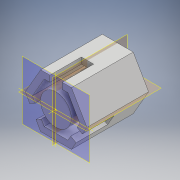
# Autodesk Inventor part: center
Saved by Autodesk Inventor 2017 (Build 210142000, 142)
## iProperties
Created: 2020-06-17
Part Number: center
Material: Generic
Document SubType Name: Modeling
Designer: HAYNIE R&D
Density: 1 g/cm^3
Appearance: Default
Author: HAYNIE R&D
Autodesk Inventor part; units mm, degrees
sketch "Sketch2" plane through (0, 0, 0) normal (0, 1, 0) x (-1, 0, 0)
  line L0 (-0.1126, -21.6377) -> (12.3874, -21.6377)
  line L1 (-0.1126, -21.6377) -> (-12.6126, -21.6377)
  line L2 (12.3874, -21.6377) -> (24.8874, 0.0129)
  line L3 (24.8874, 0.0129) -> (12.3874, 21.6635)
  line L4 (12.3874, 21.6635) -> (-12.6126, 21.6635)
  line L5 (-12.6126, 21.6635) -> (-25.1126, 0.0129)
  line L6 (-25.1126, 0.0129) -> (-12.6126, -21.6377)
  point P0 (0, 0)
  dimension "d12" = 12.5
  dimension "d13" = 12.5
  dimension "d14" = 25
  dimension "d15" = 25
  dimension "d16" = 120
  dimension "d17" = 25
  dimension "d18" = 25
  dimension "d19" = 120
  constraints: 14 end point, 3 horizontal, 1 parallel
  measures "d12" distance of L0.start L0.end
  measures "d13" distance of L0.start L1.end
  measures "d14" distance of L0.end L2.end
  measures "d15" distance of L2.end L3.end
  measures "d16" angle of L3 L2
  measures "d17" distance of L3.end L4.end
  measures "d18" distance of L4.end L5.end
  measures "d19" angle of L5 L4
extrude "Extrusion2" add sketch "Sketch2" along normal blind 50
shell "Shell1" thickness 5 removed faces 1 at (0.1126, 0, 7.2298)
sketch "Sketch3" plane through (-12.3874, 0, 21.6635) normal (0, 0, 1) x (1, 0, 0)
  line L0 (7.5, 25.4958) -> (17.5, 25.4958)
  line L1 (17.5, 25.4958) -> (17.5, -0.0042)
  line L2 (17.5, -0.0042) -> (7.5, -0.0042)
  line L3 (7.5, -0.0042) -> (7.5, 25.4958)
  line L4 (0, 0) -> (0, 50) projected
  point P0 (12.3874, 0)
  dimension "d23" = 25.5
  dimension "d24" = 10
  dimension "d25" = 7.5
  constraints: 8 end point, 2 parallel, 1 horizontal, 1 perpendicular
  measures "d23" distance of L0.end L1.end
  measures "d24" distance between parallel lines of L1 L3
  measures "d25" distance between parallel lines of L4 L3
extrude "Extrusion3" cut sketch "Sketch3" against normal blind 5
sketch "Sketch4" plane through (12.6126, 0, -21.6377) normal (0.8660254, 0, -0.5) x (-0.5, 0, -0.8660254)
  line L0 (-17.5, 25.4905) -> (-7.5, 25.4905)
  line L1 (-7.5, 25.4905) -> (-7.5, -0.0095)
  line L2 (-7.5, -0.0095) -> (-17.5, -0.0095)
  line L3 (-17.5, -0.0095) -> (-17.5, 25.4905)
  line L4 (-25, 0) -> (-25, 50) projected
  point P0 (-12.4325, 0)
  point P1 (12.3874, 0)
  dimension "d28" = 25.5
  dimension "d29" = 10
  dimension "d30" = 7.5
  constraints: 8 end point, 2 parallel, 1 horizontal, 1 perpendicular
  measures "d28" distance of L0.end L1.end
  measures "d29" distance between parallel lines of L1 L3
  measures "d30" distance between parallel lines of L3 L4
extrude "Extrusion4" cut sketch "Sketch4" against normal blind 5
sketch "Sketch5" plane through (-24.8874, 0, 0.0129) normal (-0.8660254, 0, -0.5) x (-0.5, 0, 0.8660254)
  line L0 (-17.5, 25.4996) -> (-7.5, 25.4996)
  line L1 (-7.5, 25.4996) -> (-7.5, -0.0004)
  line L2 (-7.5, -0.0004) -> (-17.5, -0.0004)
  line L3 (-17.5, -0.0004) -> (-17.5, 25.4996)
  line L4 (-25, 0) -> (-25, 50) projected
  point P0 (-12.4549, 0)
  point P1 (12.3874, 0)
  dimension "d33" = 25.5
  dimension "d34" = 10
  dimension "d35" = 7.5
  constraints: 8 end point, 2 parallel, 1 horizontal, 1 perpendicular
  measures "d33" distance of L0.end L1.end
  measures "d34" distance between parallel lines of L1 L3
  measures "d35" distance between parallel lines of L3 L4
extrude "Extrusion5" cut sketch "Sketch5" against normal blind 5
sketch "Sketch7" plane through (0, 50, 0) normal (0, 1, 0) x (1, 0, 0)
  circle A0 centre (0, 0) radius 12.5
  dimension "d39" = 25
  constraints: 1 centre point, 1 coincident
  measures "d39" diameter of A0
extrude "Extrusion6" add sketch "Sketch7" along normal blind 5 and the other way blind 50
hole "Hole1" at (-0.0018, 55, 0.0023) direction (0, -1, 0) diameter 3 depth 35 tip angle 118
body "Solid2"
